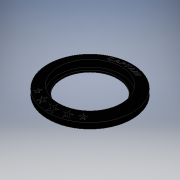
# Autodesk Inventor part: Team Pin Captain
Saved by Autodesk Inventor 2016 (Build 200138000, 138)
## iProperties
Created: 2016-02-20
Part Number: Team Pin Captain
Material: Generic
Document SubType Name: Modeling
Designer: RoksBot
Density: 1 g/cm^3
Appearance: Black
Author: RoksBot
Autodesk Inventor part; units mm, degrees
ref_plane "YZ Plane" through (0, 0, 0) normal (1, 0, 0) x (0, 1, 0)
ref_plane "XZ Plane" through (0, 0, 0) normal (0, 1, 0) x (-1, 0, 0)
ref_plane "XY Plane" through (0, 0, 0) normal (0, 0, 1) x (1, 0, 0)
sketch "Sketch1" plane through (0, 0, 0) normal (0, 0, 1) x (1, 0, 0)
  line L0 (0, 0) -> (0, 8.6646) construction
  line L1 (20.9931, 1.27) -> (20.9931, 5.715)
  line L2 (20.9931, 5.715) -> (27.9781, 3.81)
  line L3 (27.9781, 3.81) -> (27.9781, 0)
  line L4 (27.9781, 0) -> (20.9931, 0)
  line L5 (20.9931, 1.27) -> (18.4531, 1.27)
  line L6 (18.4531, 1.27) -> (18.4531, 0)
  line L7 (18.4531, 0) -> (20.9931, 0)
  dimension "d0" = 20.9931
  dimension "d1" = 4.445
  dimension "d2" = 1.27
  dimension "d3" = 2.54
  dimension "d4" = 3.81
  dimension "d5" = 6.985
  constraints: 16 end point, 2 parallel, 2 perpendicular, 2 vertical, 1 horizontal, 1 horizontal alignment
  measures "d0" distance between parallel lines of L0 L1
  measures "d1" distance from line of L5 L1.end
  measures "d2" distance of L5.end L6.end
  measures "d3" distance between parallel lines of L1 L6
  measures "d4" distance of L2.end L3.end
  measures "d5" distance between parallel lines of L1 L3
revolve "Revolution1" add sketch "Sketch1" angle 360 about axis through (0, 0, 0) along (0, 1, 0)
sketch "Sketch2" plane through (0, 1.27, 0) normal (0, 1, 0) x (1, 0, 0)
  circle A0 centre (0, 0) radius 18.4531 projected
  circle A1 centre (0, 0) radius 20.9931 projected
  circle A2 centre (0, 0) radius 27.9781 projected
  circle A3 centre (0, 0) radius 22.8981 construction
  line L0 (0.7345, -23.754) -> (1.1885, -25.1512)
  line L1 (1.1885, -25.1512) -> (0, -26.0146)
  line L2 (0, -26.0146) -> (-1.1885, -25.1512)
  line L3 (-1.1885, -25.1512) -> (-0.7345, -23.754)
  line L4 (-0.7345, -23.754) -> (0.7345, -23.754)
  line L5 (-0.7345, -23.754) -> (0, -21.4934)
  line L6 (0, -21.4934) -> (0.7345, -23.754)
  line L7 (0.7345, -23.754) -> (3.1115, -23.754)
  line L8 (3.1115, -23.754) -> (1.1885, -25.1512)
  line L9 (1.1885, -25.1512) -> (1.923, -27.4118)
  line L10 (1.923, -27.4118) -> (0, -26.0146)
  line L11 (0, -26.0146) -> (-1.923, -27.4118)
  line L12 (-1.923, -27.4118) -> (-1.1885, -25.1512)
  line L13 (-1.1885, -25.1512) -> (-3.1115, -23.754)
  line L14 (-3.1115, -23.754) -> (-0.7345, -23.754)
  line L15 (0, 0) -> (-11.4774, -31.534) construction
  line L16 (0, 0) -> (-21.0867, -27.4808) construction
  line L17 (0, 0) -> (0, -36.2985) construction
  circle A4 centre (0, 0) radius 24.765 construction
  line L18 (-8.8255, -24.2479) -> (-9.5085, -23.2352)
  line L19 (-9.5085, -23.2352) -> (-8.7565, -22.2727)
  line L20 (-8.7565, -22.2727) -> (-7.6087, -22.6905)
  line L21 (-7.6087, -22.6905) -> (-7.6514, -23.9112)
  line L22 (-7.6514, -23.9112) -> (-8.8255, -24.2479)
  line L23 (-15.5803, -20.3046) -> (-15.8569, -19.3709)
  line L24 (-15.8569, -19.3709) -> (-15.0543, -18.8193)
  line L25 (-15.0543, -18.8193) -> (-14.2817, -19.4121)
  line L26 (-14.2817, -19.4121) -> (-14.6068, -20.3301)
  line L27 (-14.6068, -20.3301) -> (-15.5803, -20.3046)
  line L28 (-15.0543, -18.8193) -> (-13.7557, -17.9267)
  line L29 (-14.2817, -19.4121) -> (-13.7557, -17.9267)
  line L30 (-14.2817, -19.4121) -> (-13.0315, -20.3714)
  line L31 (-13.0315, -20.3714) -> (-14.6068, -20.3301)
  line L32 (-14.6068, -20.3301) -> (-15.1328, -21.8155)
  line L33 (-15.5803, -20.3046) -> (-15.1328, -21.8155)
  line L34 (-15.8569, -19.3709) -> (-17.1555, -20.2634)
  line L35 (-17.1555, -20.2634) -> (-15.5803, -20.3046)
  line L36 (-15.8569, -19.3709) -> (-16.3044, -17.86)
  line L37 (-16.3044, -17.86) -> (-15.0543, -18.8193)
  line L38 (-8.7565, -22.2727) -> (-7.5398, -20.7153)
  line L39 (-7.6087, -22.6905) -> (-7.5398, -20.7153)
  line L40 (-7.6514, -23.9112) -> (-5.7515, -23.3664)
  line L41 (-5.7515, -23.3664) -> (-7.6087, -22.6905)
  line L42 (-7.6514, -23.9112) -> (-7.7203, -25.8863)
  line L43 (-7.7203, -25.8863) -> (-8.8255, -24.2479)
  line L44 (-8.8255, -24.2479) -> (-10.7253, -24.7926)
  line L45 (-10.7253, -24.7926) -> (-9.5085, -23.2352)
  line L46 (-9.5085, -23.2352) -> (-10.6137, -21.5967)
  line L47 (-10.6137, -21.5967) -> (-8.7565, -22.2727)
  line L48 (8.8255, -24.2479) -> (9.5085, -23.2352)
  line L49 (9.5085, -23.2352) -> (8.7565, -22.2727)
  line L50 (8.7565, -22.2727) -> (7.6087, -22.6905)
  line L51 (7.6087, -22.6905) -> (7.6514, -23.9112)
  line L52 (7.6514, -23.9112) -> (8.8255, -24.2479)
  line L53 (15.5803, -20.3046) -> (15.8569, -19.3709)
  line L54 (15.8569, -19.3709) -> (15.0543, -18.8193)
  line L55 (15.0543, -18.8193) -> (14.2817, -19.4121)
  line L56 (14.2817, -19.4121) -> (14.6068, -20.3301)
  line L57 (14.6068, -20.3301) -> (15.5803, -20.3046)
  line L58 (15.0543, -18.8193) -> (13.7557, -17.9267)
  line L59 (14.2817, -19.4121) -> (13.7557, -17.9267)
  line L60 (13.0315, -20.3714) -> (14.6068, -20.3301)
  line L61 (14.6068, -20.3301) -> (15.1328, -21.8155)
  line L62 (15.5803, -20.3046) -> (15.1328, -21.8155)
  line L63 (15.8569, -19.3709) -> (17.1555, -20.2634)
  line L64 (17.1555, -20.2634) -> (15.5803, -20.3046)
  line L65 (15.8569, -19.3709) -> (16.3044, -17.86)
  line L66 (16.3044, -17.86) -> (15.0543, -18.8193)
  line L67 (8.7565, -22.2727) -> (7.5398, -20.7153)
  line L68 (7.6087, -22.6905) -> (7.5398, -20.7153)
  line L69 (7.6514, -23.9112) -> (5.7515, -23.3664)
  line L70 (5.7515, -23.3664) -> (7.6087, -22.6905)
  line L71 (7.6514, -23.9112) -> (7.7203, -25.8863)
  line L72 (7.7203, -25.8863) -> (8.8255, -24.2479)
  line L73 (8.8255, -24.2479) -> (10.7253, -24.7926)
  line L74 (10.7253, -24.7926) -> (9.5085, -23.2352)
  line L75 (9.5085, -23.2352) -> (10.6137, -21.5967)
  line L76 (10.6137, -21.5967) -> (8.7565, -22.2727)
  line L77 (14.2817, -19.4121) -> (13.0315, -20.3714)
  spline S0 degree 2 poles (-7.452, 22.2728) (-7.5894, 21.8382) (-7.999, 21.383) (-8.3584, 21.2408) knots 0 0 0 1 2 2 2
  spline S1 degree 2 poles (-8.3584, 21.2408) (-8.9714, 20.9984) (-9.5636, 21.3634) knots 0 0 0 1 1 1
  spline S2 degree 2 poles (-9.5636, 21.3634) (-10.1692, 21.7296) (-10.5043, 22.5766) knots 0 0 0 1 1 1
  spline S3 degree 2 poles (-10.5043, 22.5766) (-10.8746, 23.5128) (-10.62, 24.1806) knots 0 0 0 1 1 1
  spline S4 degree 2 poles (-10.62, 24.1806) (-10.4159, 24.7156) (-9.8977, 24.9206) knots 0 0 0 1 1 1
  spline S5 degree 2 poles (-9.8977, 24.9206) (-9.4937, 25.0804) (-9.2123, 25.0531) knots 0 0 0 1 1 1
  spline S6 degree 2 poles (-9.2123, 25.0531) (-8.9003, 25.0219) (-8.588, 24.762) knots 0 0 0 1 1 1
  spline S7 degree 2 poles (-8.588, 24.762) (-8.5215, 24.7077) (-8.4961, 24.6437) knots 0 0 0 1 1 1
  spline S8 degree 2 poles (-8.4961, 24.6437) (-8.452, 24.5322) (-8.5586, 24.3129) (-8.6617, 24.2721) knots 0 0 0 1 2 2 2
  spline S9 degree 2 poles (-8.6617, 24.2721) (-8.8066, 24.2148) (-8.9519, 24.3377) knots 0 0 0 1 1 1
  spline S10 degree 2 poles (-8.9519, 24.3377) (-9.1105, 24.4619) (-9.2997, 24.4676) knots 0 0 0 1 1 1
  spline S11 degree 2 poles (-9.2997, 24.4676) (-9.4454, 24.4776) (-9.6878, 24.3817) knots 0 0 0 1 1 1
  spline S12 degree 2 poles (-9.6878, 24.3817) (-10.0026, 24.2572) (-10.1086, 23.8898) knots 0 0 0 1 1 1
  spline S13 degree 2 poles (-10.1086, 23.8898) (-10.2417, 23.4441) (-9.9805, 22.7838) knots 0 0 0 1 1 1
  spline S14 degree 2 poles (-9.9805, 22.7838) (-9.7402, 22.1764) (-8.9417, 21.632) (-8.5628, 21.7819) knots 0 0 0 1 2 2 2
  spline S15 degree 2 poles (-8.5628, 21.7819) (-8.1532, 21.9439) (-7.9982, 22.4563) knots 0 0 0 1 1 1
  spline S16 degree 2 poles (-7.9982, 22.4563) (-7.9577, 22.5819) (-7.8379, 22.6293) knots 0 0 0 1 1 1
  spline S17 degree 2 poles (-7.8379, 22.6293) (-7.7348, 22.67) (-7.497, 22.574) (-7.454, 22.4653) knots 0 0 0 1 2 2 2
  spline S18 degree 2 poles (-7.454, 22.4653) (-7.4188, 22.3762) (-7.452, 22.2728) knots 0 0 0 1 1 1
  spline S19 degree 2 poles (-4.0032, 22.9542) (-3.9599, 22.8874) (-3.9484, 22.8378) knots 0 0 0 1 1 1
  spline S20 degree 2 poles (-3.9484, 22.8378) (-3.9211, 22.7211) (-4.0602, 22.5256) (-4.174, 22.4991) knots 0 0 0 1 2 2 2
  spline S21 degree 2 poles (-4.174, 22.4991) (-4.3519, 22.4576) (-4.4614, 22.6105) knots 0 0 0 1 1 1
  line L78 (-4.4614, 22.6105) -> (-4.7037, 22.9632)
  line L79 (-4.7037, 22.9632) -> (-5.9467, 22.6734)
  line L80 (-5.9467, 22.6734) -> (-6.0023, 22.2389)
  spline S22 degree 2 poles (-6.0023, 22.2389) (-6.0297, 22.0664) (-6.2136, 22.0235) knots 0 0 0 1 1 1
  spline S23 degree 2 poles (-6.2136, 22.0235) (-6.3215, 21.9983) (-6.5313, 22.1063) (-6.5585, 22.223) knots 0 0 0 1 2 2 2
  spline S24 degree 2 poles (-6.5585, 22.223) (-6.5701, 22.2726) (-6.5635, 22.3234) knots 0 0 0 1 1 1
  line L81 (-6.5635, 22.3234) -> (-6.1883, 25.2137)
  spline S25 degree 2 poles (-6.1883, 25.2137) (-6.1105, 25.3948) (-5.9588, 25.4302) knots 0 0 0 1 1 1
  spline S26 degree 2 poles (-5.9588, 25.4302) (-5.7983, 25.4676) (-5.6521, 25.3418) knots 0 0 0 1 1 1
  line L82 (-5.6521, 25.3418) -> (-4.0032, 22.9542)
  line L83 (-5.0075, 23.4615) -> (-5.7381, 24.5495)
  line L84 (-5.7381, 24.5495) -> (-5.8975, 23.254)
  line L85 (-5.8975, 23.254) -> (-5.0075, 23.4615)
  spline S27 degree 2 poles (-1.4128, 25.1706) (-1.373, 24.7801) (-1.7405, 24.2487) (-2.1221, 24.2099) knots 0 0 0 1 2 2 2
  line L86 (-2.1221, 24.2099) -> (-2.8613, 24.1346)
  line L87 (-2.8613, 24.1346) -> (-2.7435, 22.9781)
  spline S28 degree 2 poles (-2.7435, 22.9781) (-2.7141, 22.6889) (-2.9883, 22.661) knots 0 0 0 1 1 1
  spline S29 degree 2 poles (-2.9883, 22.661) (-3.2655, 22.6328) (-3.295, 22.9219) knots 0 0 0 1 1 1
  line L88 (-3.295, 22.9219) -> (-3.594, 25.858)
  line L89 (-3.594, 25.858) -> (-2.3689, 25.9827)
  spline S30 degree 2 poles (-2.3689, 25.9827) (-1.5044, 26.0708) (-1.4128, 25.1706) knots 0 0 0 1 1 1
  spline S31 degree 2 poles (-1.9642, 25.1144) (-1.9979, 25.4453) (-2.3109, 25.4134) knots 0 0 0 1 1 1
  line L90 (-2.3109, 25.4134) -> (-2.9845, 25.3448)
  line L91 (-2.9845, 25.3448) -> (-2.9193, 24.7039)
  line L92 (-2.9193, 24.7039) -> (-2.18, 24.7792)
  spline S32 degree 2 poles (-2.18, 24.7792) (-1.9326, 24.8044) (-1.9642, 25.1144) knots 0 0 0 1 1 1
  line L93 (1.4886, 25.4732) -> (0.8176, 25.4852)
  line L94 (0.8176, 25.4852) -> (0.7753, 23.1336)
  spline S33 degree 2 poles (0.7753, 23.1336) (0.7699, 22.831) (0.4733, 22.8364) knots 0 0 0 1 1 1
  spline S34 degree 2 poles (0.4733, 22.8364) (0.1767, 22.8417) (0.1822, 23.1443) knots 0 0 0 1 1 1
  line L95 (0.1822, 23.1443) -> (0.2244, 25.4959)
  line L96 (0.2244, 25.4959) -> (-0.4466, 25.5079)
  spline S35 degree 2 poles (-0.4466, 25.5079) (-0.7432, 25.5133) (-0.7378, 25.8128) knots 0 0 0 1 1 1
  spline S36 degree 2 poles (-0.7378, 25.8128) (-0.7325, 26.1064) (-0.436, 26.1011) knots 0 0 0 1 1 1
  line L97 (-0.436, 26.1011) -> (1.4993, 26.0663)
  spline S37 degree 2 poles (1.4993, 26.0663) (1.8018, 26.0609) (1.7966, 25.7673) knots 0 0 0 1 1 1
  spline S38 degree 2 poles (1.7966, 25.7673) (1.7912, 25.4677) (1.4886, 25.4732) knots 0 0 0 1 1 1
  spline S39 degree 2 poles (4.8349, 22.7936) (4.8501, 22.7154) (4.8424, 22.6651) knots 0 0 0 1 1 1
  spline S40 degree 2 poles (4.8424, 22.6651) (4.8242, 22.5466) (4.6224, 22.417) (4.5069, 22.4348) knots 0 0 0 1 2 2 2
  spline S41 degree 2 poles (4.5069, 22.4348) (4.3262, 22.4626) (4.2816, 22.6453) knots 0 0 0 1 1 1
  line L98 (4.2816, 22.6453) -> (4.1881, 23.0628)
  line L99 (4.1881, 23.0628) -> (2.9266, 23.2568)
  line L100 (2.9266, 23.2568) -> (2.7132, 22.8743)
  spline S42 degree 2 poles (2.7132, 22.8743) (2.6234, 22.7244) (2.4369, 22.7531) knots 0 0 0 1 1 1
  spline S43 degree 2 poles (2.4369, 22.7531) (2.3273, 22.77) (2.1728, 22.9483) (2.1911, 23.0668) knots 0 0 0 1 2 2 2
  spline S44 degree 2 poles (2.1911, 23.0668) (2.1988, 23.1171) (2.2239, 23.1618) knots 0 0 0 1 1 1
  line L101 (2.2239, 23.1618) -> (3.6486, 25.7043)
  spline S45 degree 2 poles (3.6486, 25.7043) (3.7882, 25.8435) (3.9422, 25.8198) knots 0 0 0 1 1 1
  spline S46 degree 2 poles (3.9422, 25.8198) (4.1051, 25.7948) (4.1939, 25.6235) knots 0 0 0 1 1 1
  line L102 (4.1939, 25.6235) -> (4.8349, 22.7936)
  line L103 (4.0918, 23.6384) -> (3.819, 24.9202)
  line L104 (3.819, 24.9202) -> (3.1885, 23.7773)
  line L105 (3.1885, 23.7773) -> (4.0918, 23.6384)
  spline S47 degree 2 poles (6.0974, 22.3337) (6.0238, 22.0525) (5.7485, 22.1246) knots 0 0 0 1 1 1
  spline S48 degree 2 poles (5.7485, 22.1246) (5.4731, 22.1967) (5.5467, 22.4778) knots 0 0 0 1 1 1
  line L106 (5.5467, 22.4778) -> (6.2195, 25.0489)
  spline S49 degree 2 poles (6.2195, 25.0489) (6.2924, 25.3271) (6.5677, 25.2551) knots 0 0 0 1 1 1
  spline S50 degree 2 poles (6.5677, 25.2551) (6.8431, 25.183) (6.7703, 24.9047) knots 0 0 0 1 1 1
  line L107 (6.7703, 24.9047) -> (6.0974, 22.3337)
  spline S51 degree 2 poles (9.0693, 21.3296) (8.9667, 21.0513) (8.7362, 21.1362) knots 0 0 0 1 1 1
  spline S52 degree 2 poles (8.7362, 21.1362) (8.5816, 21.1932) (8.5366, 21.4524) knots 0 0 0 1 1 1
  line L108 (8.5366, 21.4524) -> (8.0179, 23.7541)
  line L109 (8.0179, 23.7541) -> (7.355, 21.9548)
  spline S53 degree 2 poles (7.355, 21.9548) (7.2545, 21.6821) (6.9931, 21.7784) knots 0 0 0 1 1 1
  spline S54 degree 2 poles (6.9931, 21.7784) (6.7316, 21.8747) (6.8321, 22.1474) knots 0 0 0 1 1 1
  line L110 (6.8321, 22.1474) -> (7.759, 24.6637)
  spline S55 degree 2 poles (7.759, 24.6637) (7.8564, 24.928) (8.1094, 24.8348) knots 0 0 0 1 1 1
  spline S56 degree 2 poles (8.1094, 24.8348) (8.2612, 24.7788) (8.2231, 24.6492) knots 0 0 0 1 1 1
  line L111 (8.2231, 24.6492) -> (8.8177, 22.2589)
  line L112 (8.8177, 22.2589) -> (9.4629, 24.0105)
  spline S57 degree 2 poles (9.4629, 24.0105) (9.5624, 24.2804) (9.8238, 24.184) knots 0 0 0 1 1 1
  spline S58 degree 2 poles (9.8238, 24.184) (10.0853, 24.0877) (9.9859, 23.8178) knots 0 0 0 1 1 1
  line L113 (9.9859, 23.8178) -> (9.0693, 21.3296)
  point P0 (0, -24.765)
  point P1 (-8.4701, -23.2715)
  point P2 (-15.076, -19.6474)
  point P3 (8.4701, -23.2715)
  point P4 (15.076, -19.6474)
  dimension "d7" = 1.905
  dimension "d10" = 6.223
  dimension "d11" = 20
  dimension "d12" = 17.5
  dimension "d13" = 49.53
  dimension "d14" = 2.2606
  dimension "d15" = 1.8796
  dimension "d16" = 1.4986
  dimension "d19" = 1.8796
  dimension "d20" = 1.4986
  constraints: 156 end point, 27 collinear, 24 symmetric about line, 11 point on line, 3 point on circle, 2 centre point, 2 coincident, 2 horizontal, 1 vertical, 1 vertical alignment, 34 other
  measures "d7" radial gap between concentric circles of A1 A3
  measures "d10" distance of L9.end L5.end
  measures "d11" angle of L17 L15
  measures "d12" angle of L15 L16
  measures "d13" diameter of A4
  measures "d14" distance from line of L1.end L4
  measures "d15" distance from line of L18.start L20
  measures "d16" distance from line of L23.start L25
  measures "d19" distance from line of L48.start L50
  measures "d20" distance from line of L62.start L55
extrude "Extrusion1" cut sketch "Sketch2" along normal through all contours L7 L8 L0 | L0 L1 L2 L3 L4 | L4 L5 L6 | L9 L10 L1 | L3 L13 L14 | L11 L12 L2 | L44 L45 L18 | L18 L19 L20 L21 L22 | L22 L42 L43 | L46 L47 L19 | L21 L41 L40 | L38 L39 L20 | L35 L34 L23 | L23 L24 L25 L26 L27 | L27 L32 L33 | L36 L37 L24 | L26 L30 L31 | L28 L29 L25 | L52 L51 L50 L49 L48 | L72 L71 L52 | L48 L74 L73 | L49 L76 L75 | L69 L70 L51 | L50 L68 L67 | L57 L56 L55 L54 L53 | L62 L61 L57 | L53 L63 L64 | L54 L66 L65 | L60 L77 L56 | L55 L59 L58 | S0 S1 S2 S3 S4 S5 S6 S7 S8 S9 S10 S11 S12 S13 S14 S15 S16 S17 S18 | S19 S20 S21 L78 L79 L80 S22 S23 S24 L81 S25 S26 L82 | S27 L86 L87 S28 S29 L88 L89 S30 | L93 L94 S33 S34 L95 L96 S35 S36 L97 S37 S38 | S39 S40 S41 L98 L99 L100 S42 S43 S44 L101 S45 S46 L102 | S47 S48 L106 S49 S50 L107 | S51 S52 L108 L109 S53 S54 L110 S55 S56 L111 L112 S57 S58 L113
body "Solid1"
